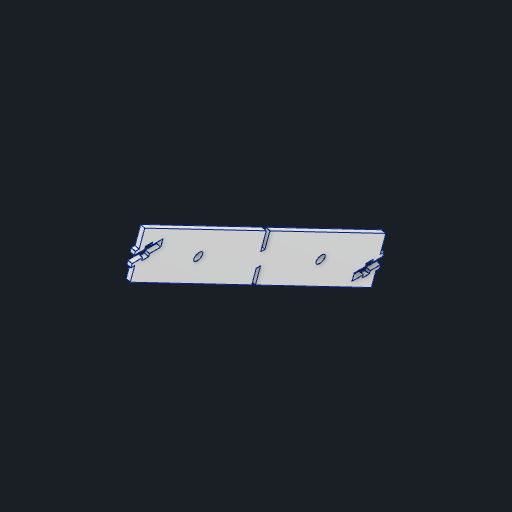
# Autodesk Inventor part: SidePlate
Saved by Autodesk Inventor 2023 (Build 270158000, 158)
## iProperties
Created: 2022-06-19
Part Number: SidePlate
Material: Aluminum 6061
Document SubType Name: Modeling
Designer: FizzyApple12
Density: 2.7 g/cm^3
Appearance: Aluminum - Flat
Author: FizzyApple12
Autodesk Inventor part; units mm, degrees
ref_plane "YZ Plane" through (0, 0, 0) normal (1, 0, 0) x (0, 1, 0)
ref_plane "XZ Plane" through (0, 0, 0) normal (0, 1, 0) x (-1, 0, 0)
ref_plane "Work Plane1" through (111.7581, 40.3852, 111.4201) normal (-0.9659258, 0.258819, 0) x (-0.1358803, -0.507112, -0.8511016)
sketch "Sketch1" plane through (111.7581, 40.3852, 111.4201) normal (-0.9659258, 0.258819, 0) x (-0.1358803, -0.507112, -0.8511016)
  line L0 (0, -6.3437) -> (253.9995, -6.3437) construction
  line L1 (228.4809, -42.564) -> (250.8233, -6.3437) construction
  line L2 (108.9501, -41.6524) -> (130.3466, -6.9656) construction
  line L3 (107.0353, -38.7089) -> (126.9998, -6.3437) construction
  line L4 (-20.5605, -41.6524) -> (-3.3186, -13.7009) construction
  line L5 (-4.9348, -10.2733) -> (-23.2434, -39.9543) construction
  line L6 (-3.3186, -13.7009) -> (1.2196, -6.3437) construction
  line L7 (130.3466, -6.9656) -> (130.7302, -6.3437) construction
  line L8 (130.7302, -6.3437) -> (250.8233, -6.3437)
  line L9 (126.9998, -6.3437) -> (1.2196, -6.3437)
  line L10 (-20.5605, -41.6524) -> (108.9501, -41.6524) construction
  line L11 (108.9501, -41.6524) -> (232.7736, -41.6524) construction
  line L12 (107.0353, -38.7089) -> (105.2196, -41.6524) construction
  line L13 (229.0432, -41.6524) -> (250.8233, -6.3437)
  line L14 (229.0432, -41.6524) -> (108.9501, -41.6524)
  line L15 (130.7302, -6.3437) -> (108.9501, -41.6524)
  line L16 (105.2196, -41.6524) -> (126.9998, -6.3437)
  line L17 (105.2196, -41.6524) -> (-20.5605, -41.6524)
  line L18 (-20.5605, -41.6524) -> (1.2196, -6.3437)
  line L19 (120.3322, -17.1527) -> (123.0345, -18.8196)
  line L20 (113.6647, -27.9617) -> (116.367, -29.6286)
  line L21 (244.1558, -17.1527) -> (246.8581, -18.8196)
  line L22 (246.8581, -18.8196) -> (240.1905, -29.6286)
  line L23 (240.1905, -29.6286) -> (237.4883, -27.9617)
  line L24 (-5.4479, -17.1527) -> (-8.1501, -15.4858)
  line L25 (-8.1501, -15.4858) -> (-14.8176, -26.2948)
  line L26 (-14.8176, -26.2948) -> (-12.1154, -27.9617)
  line L27 (256.5554, -3.0988) -> (232.2107, -42.5651) construction
  line L28 (105.2196, -41.6524) -> (134.1991, 5.3274) construction
  line L29 (136.9013, 3.6606) -> (107.9219, -43.3193) construction
  line L30 (12.8127, 12.4503) -> (-20.8503, -42.1222) construction
  line L31 (-23.5525, -40.4553) -> (10.1104, 14.1172) construction
  line L32 (256.5554, -3.0988) -> (232.2107, -42.5651) construction
  line L33 (237.4883, -27.9617) -> (229.5084, -40.8982) construction
  line L34 (250.8233, -6.3437) -> (244.1558, -17.1527) construction
  point P0 (126.9998, -6.3437)
  dimension "d0" = 12.7
  dimension "d1" = 12.7
  dimension "d2" = 12.7
  dimension "d3" = 12.7
  dimension "d4" = 12.7
  dimension "d5" = 12.7
  constraints: 52 end point, 25 point on line, 12 collinear, 6 perpendicular, 3 parallel, 1 midpoint
  measures "d0" distance between parallel lines of L19 L20
  measures "d1" distance from line of point (127, -6.344) L19
  measures "d2" distance of L21.end L22.end
  measures "d3" distance from line of L1.end L21
  measures "d4" distance of L24.end L25.end
  measures "d5" distance from line of L6.end L24
extrude "Extrusion1" add sketch "Sketch1" along normal blind 3.175
sketch "Sketch2" plane through (111.7581, 40.3852, 111.4201) normal (0.9659258, -0.258819, 0) x (-0.1358803, -0.507112, -0.8511016)
  line L0 (-20.5605, 41.6524) -> (105.2196, 41.6524) construction
  line L1 (42.3296, 41.6524) -> (64.1097, 6.3437) construction
  line L2 (126.9998, 6.3437) -> (1.2196, 6.3437) construction
  line L3 (108.9501, 41.6524) -> (229.0432, 41.6524) construction
  line L4 (168.9966, 41.6524) -> (190.7768, 6.3437) construction
  line L5 (250.8233, 6.3437) -> (130.7302, 6.3437) construction
  point P0 (130.4954, 0.6768)
  point P1 (53.2196, 23.9981)
  point P2 (179.8867, 23.9981)
  constraints: 6 midpoint, 4 end point
hole "Hole1" at (109.8129, 33.1257, 53.5258) at (92.6013, -31.1087, -54.2807) direction (-0.9659258, 0.258819, 0) diameter 6.7564 depth 13.6144 clearance for "Flat Head Machine Screw (82)" size "1/4" standard "Ansi Unified Screw Threads"
sketch "Sketch3" plane through (111.7581, 40.3852, 111.4201) normal (0.9659258, -0.258819, 0) x (-0.1358803, -0.507112, -0.8511016)
  line L0 (-8.1501, 15.4858) -> (-14.8176, 26.2948) projected
  line L1 (-11.4839, 20.8903) -> (6.8914, 32.2251) construction
  line L2 (5.2245, 34.9273) -> (-13.1507, 23.5925)
  line L3 (-8.1501, 15.4858) -> (-14.8176, 26.2948) projected
  line L4 (-9.817, 18.1881) -> (8.5583, 29.5228)
  line L5 (2.7826, 23.1623) -> (-3.0515, 32.6201)
  line L6 (-3.0515, 32.6201) -> (-7.3751, 29.9531)
  line L7 (-7.3751, 29.9531) -> (-1.541, 20.4953)
  line L8 (-1.541, 20.4953) -> (2.7826, 23.1623)
  line L9 (-7.3751, 29.9531) -> (2.7826, 23.1623) construction
  line L10 (240.1905, 29.6286) -> (246.8581, 18.8196) projected
  line L11 (243.5243, 24.2241) -> (225.149, 12.8893) construction
  line L12 (5.2245, 34.9273) -> (8.5583, 29.5228)
  line L13 (223.4821, 15.5915) -> (226.8159, 10.187)
  line L14 (226.8159, 10.187) -> (245.1912, 21.5218)
  line L15 (223.4821, 15.5915) -> (241.8574, 26.9263)
  line L16 (239.4155, 15.1612) -> (235.0919, 12.4942)
  line L17 (235.0919, 12.4942) -> (229.2578, 21.9521)
  line L18 (229.2578, 21.9521) -> (233.5814, 24.6191)
  line L19 (233.5814, 24.6191) -> (239.4155, 15.1612)
  line L20 (239.4155, 15.1612) -> (229.2578, 21.9521) construction
  line L21 (-14.4934, 26.4948) -> (-7.8258, 15.6858)
  line L22 (-14.8176, 26.2948) -> (-12.1154, 27.9617) projected
  line L23 (-5.4479, 17.1527) -> (-8.1501, 15.4858) projected
  line L24 (239.8663, 29.4285) -> (246.584, 18.5381)
  line L25 (246.8581, 18.8196) -> (244.1558, 17.1527) projected
  line L26 (237.4883, 27.9617) -> (240.1905, 29.6286) projected
  point P0 (130.4954, 0.6768)
  point P1 (-2.2962, 26.5577)
  point P2 (234.3367, 18.5567)
  point P3 (1.5325, 25.1889)
  point P4 (-1.8013, 30.5934)
  point P5 (-6.1249, 27.9264)
  point P6 (-9.817, 18.1881)
  point P7 (-2.7911, 22.5219)
  point P8 (238.1653, 17.1879)
  point P9 (234.8316, 22.5924)
  point P10 (230.508, 19.9254)
  point P11 (233.8417, 14.5209)
  point P12 (241.5332, 26.7263)
  point P13 (246.5338, 18.6195)
  point P14 (244.8669, 21.3218)
  point P15 (-12.8265, 23.7926)
  point P16 (-9.4927, 18.3881)
  dimension "d16" = 21.59
  dimension "d19" = 11.1125
  dimension "d20" = 5.08
  dimension "d21" = 21.59
  dimension "d22" = 6.35
  dimension "d23" = 6.35
  dimension "d24" = 5.08
  dimension "d25" = 11.1125
  dimension "d28" = 0.381
  dimension "d29" = 0.381
  constraints: 40 end point, 10 perpendicular, 8 midpoint, 8 parallel, 7 point on line
  measures "d16" distance of L1.end L1.start
  measures "d19" distance of L5.start L5.end
  measures "d20" distance of L5.end L6.end
  measures "d21" distance of L11.end L11.start
  measures "d22" distance of L2.start L4.end
  measures "d23" distance of L13.start L13.end
  measures "d24" distance between parallel lines of L17 L19
  measures "d25" distance between parallel lines of L18 L16
  measures "d28" distance between parallel lines of L0 L21
  measures "d29" distance between parallel lines of L10 L24
extrude "Extrusion2" cut sketch "Sketch3" against normal through all
body "Solid1"
